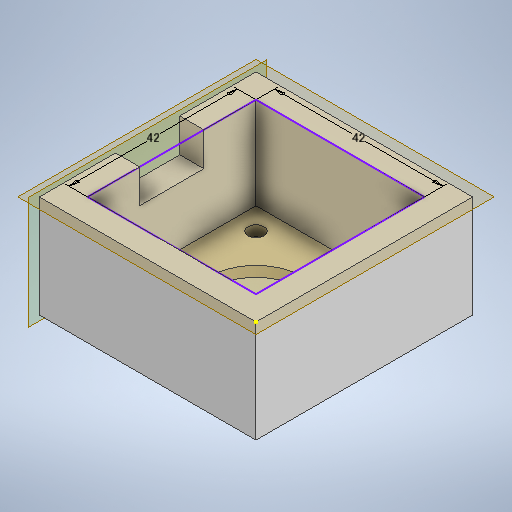
# Autodesk Inventor part: motor_case
Saved by Autodesk Inventor 2025.1 (Build 291241000, 241)
## iProperties
Created: 2024-11-24
Part Number: motor_case
Material: 一般
Document SubType Name: Modeling
Designer: dell
Density: 1 g/cm^3
Appearance: 既定
Author: dell
Autodesk Inventor part; units mm, degrees
ref_plane "YZ Plane" through (0, 0, 0) normal (1, 0, 0) x (0, 1, 0)
ref_plane "XZ Plane" through (0, 0, 0) normal (0, 1, 0) x (-1, 0, 0)
ref_plane "XY Plane" through (0, 0, 0) normal (0, 0, 1) x (1, 0, 0)
sketch "スケッチ1" plane through (0, 0, 0) normal (0, 1, 0) x (-1, 0, 0)
  line L0 (0, 0) -> (54, 0)
  line L1 (54, 0) -> (54, -54)
  line L2 (54, -54) -> (0, -54)
  line L3 (0, -54) -> (0, 0)
  dimension "d0" = 54
  dimension "d1" = 54
  constraints: 8 end point, 2 parallel, 1 horizontal, 1 perpendicular
  measures "d0" distance of L0.end L1.end
  measures "d1" distance of L1.end L2.end
extrude "押し出し1" add sketch "スケッチ1" along normal blind 25.5
ref_plane "作業平面1" through (0, 25.5, 0) normal (0, 1, 0) x (1, 0, 0)
sketch "スケッチ2" plane through (0, 25.5, 0) normal (0, 1, 0) x (1, 0, 0)
  line L0 (-6, 6) -> (-48, 6)
  line L1 (-48, 6) -> (-48, 48)
  line L2 (-48, 48) -> (-6, 48)
  line L3 (-6, 48) -> (-6, 6)
  point P0 (0, 0)
  dimension "d5" = 42
  dimension "d6" = 42
  constraints: 8 end point, 2 parallel, 1 horizontal, 1 perpendicular
  measures "d5" distance of L1.end L2.end
  measures "d6" distance of L0.end L1.end
shell "シェル1" thickness 6 removed faces 1 at (-36, 25.5, -36) ; own thickness 2.6 on faces at (-36, 0, -36)
ref_plane "作業平面2" through (-48, 2.6, -48) normal (0, 1, 0) x (1, 0, 0)
sketch "スケッチ3" plane through (-48, 2.6, -48) normal (0, 1, 0) x (1, 0, 0)
  line L0 (0, 0) -> (42, 0) projected
  line L1 (0, -42) -> (0, 0) projected
  line L2 (42, 0) -> (42, -42) projected
  line L3 (42, -42) -> (0, -42) projected
  point P0 (48, -48)
  point P1 (5.5, -5.5)
  point P2 (36.5, -5.5)
  point P3 (36.5, -36.5)
  point P4 (5.5, -36.5)
  dimension "d10" = 5.5
  dimension "d11" = 5.5
  dimension "d12" = 5.5
  dimension "d13" = 5.5
  dimension "d14" = 5.5
  dimension "d15" = 5.5
  dimension "d16" = 5.5
  dimension "d17" = 5.5
  measures "d10" distance from line of L0 point (5.5, -5.5)
  measures "d11" distance from line of L1 point (5.5, -5.5)
  measures "d12" distance from line of L0 point (36.5, -5.5)
  measures "d13" distance from line of L2 point (36.5, -5.5)
  measures "d14" distance from line of L2 point (36.5, -36.5)
  measures "d15" distance from line of L3 point (36.5, -36.5)
  measures "d16" distance from line of L3 point (5.5, -36.5)
  measures "d17" distance from line of L1 point (5.5, -36.5)
hole "穴1" at (-11.5, 2.6, -42.5) at (-11.5, 2.6, -11.5) at (-42.5, 2.6, -42.5) at (-42.5, 2.6, -11.5) direction (0, -1, 0) diameter 4 end through all
sketch "スケッチ4" plane through (-48, 2.6, -48) normal (0, 1, 0) x (1, 0, 0)
  point P0 (48, -48)
  point P1 (21, -21)
hole "穴2" at (-27, 2.6, -27) direction (0, -1, 0) diameter 23 end through all
ref_plane "作業平面3" through (-54, 0, -54) normal (-1, 0, 0) x (0, 0, 1)
sketch "スケッチ5" plane through (-54, 0, -54) normal (-1, 0, 0) x (0, 0, 1)
  line L0 (0, 25.5) -> (54, 25.5) projected
  line L1 (0, 0) -> (54, 0) projected
  line L2 (35, 25.5) -> (19, 25.5)
  line L3 (19, 25.5) -> (19, 17.1)
  line L4 (19, 17.1) -> (35, 17.1)
  line L5 (35, 17.1) -> (35, 25.5)
  point P0 (27, 25.5)
  point P1 (27, 25.5)
  point P2 (19, 25.5)
  dimension "d33" = 16
  dimension "d34" = 8.4
  dimension "d35" = 8
  constraints: 8 end point, 2 midpoint, 2 parallel, 1 horizontal, 1 perpendicular, 1 point on line
  measures "d33" distance of L4.end L3.end
  measures "d34" distance of L2.end L3.end
  measures "d35" distance of L2.end point (27, 25.5)
extrude "押し出し2" cut sketch "スケッチ5" against normal blind 6
